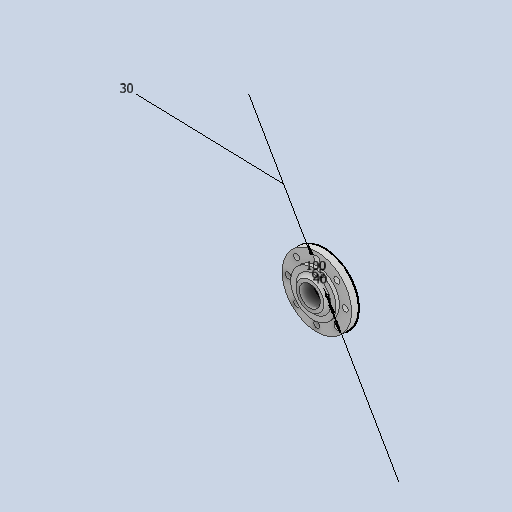
# Autodesk Inventor part: Part11_CPY
Saved by Autodesk Inventor 2023 (Build 270158000, 158)
## iProperties
Created: 2023-01-29
Part Number: Part11_CPY
Material: Generic
Document SubType Name: Modeling
Designer: Merve Babacan
Density: 1 g/cm^3
Appearance: Default
Author: Merve Babacan
Autodesk Inventor part; units mm, degrees
ref_plane "YZ Plane" through (0, 0, 0) normal (1, 0, 0) x (0, 1, 0)
ref_plane "XZ Plane" through (0, 0, 0) normal (0, 1, 0) x (-1, 0, 0)
ref_plane "XY Plane" through (0, 0, 0) normal (0, 0, 1) x (1, 0, 0)
sketch "Sketch1" plane through (0, 0, 0) normal (0, 0, 1) x (1, 0, 0)
  circle A0 centre (0, 0) radius 15
  circle A1 centre (0, 0) radius 20
  circle A2 centre (0, 0) radius 32.5
  circle A3 centre (0, 0) radius 50
  dimension "d0" = 30
  dimension "d1" = 40
  dimension "d2" = 65
  dimension "d3" = 100
  constraints: 4 centre point, 4 coincident
  measures "d0" diameter of A0
  measures "d1" diameter of A1
  measures "d2" diameter of A2
  measures "d3" diameter of A3
extrude "Extrusion1" add sketch "Sketch1" along normal blind 10 contours A2 | A3
extrude "Extrusion2" add sketch "Sketch1" along normal blind 20 contours A1
extrude "Extrusion3" add sketch "Sketch1" along normal blind 15 contours A2
fillet "Fillet1" radius 5 1 edges at (-20, 0, 15)
extrude "Extrusion4" add sketch "Sketch1" against normal blind 2 contours A1 | A2
sketch "Sketch2" plane through (0, 0, 10) normal (0, 0, 1) x (1, 0, 0)
  point P0 (0, 0)
  point P1 (0, 41)
  point P2 (28.9914, 28.9914)
  point P3 (41, 0)
  point P4 (28.9914, -28.9914)
  point P5 (0, -41)
  point P6 (-28.9914, -28.9914)
  point P7 (-41, 0)
  point P8 (-28.9914, 28.9914)
  dimension "d13" = 41
  dimension "d16" = 360
  constraints: 9 other
  measures "d13" distance of point (0, 0) point (0, 41)
hole "Hole1" at (0, 41, 10) at (28.9914, 28.9914, 10) at (41, 0, 10) at (28.9914, -28.9914, 10) at (0, -41, 10) at (-28.9914, -28.9914, 10) at (-41, 0, 10) at (-28.9914, 28.9914, 10) direction (0, 0, -1) diameter 8.5 depth 26 tip angle 118
body "Solid1"
